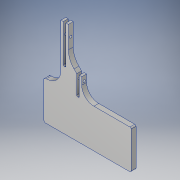
# Autodesk Inventor part: 2BarClawPaddle
Saved by Autodesk Inventor 2017 (Build 210142000, 142)
## iProperties
Created: 2017-09-30
Part Number: 2BarClawPaddle
Material: Aluminum 6061
Document SubType Name: Modeling
Designer: User
Density: 2.7 g/cm^3
Appearance: Aluminum - Flat
Mass: 78.5401 g
Surface Area: 128.456 cm^2
Volume: 29.0889 cm^3
Author: User
Autodesk Inventor part; units mm, degrees
ref_plane "YZ Plane" through (0, 0, 0) normal (1, 0, 0) x (0, 1, 0)
ref_plane "XZ Plane" through (0, 0, 0) normal (0, 1, 0) x (-1, 0, 0)
ref_plane "XY Plane" through (0, 0, 0) normal (0, 0, 1) x (1, 0, 0)
sketch "Sketch1" plane through (0, 0, 0) normal (0, 0, 1) x (1, 0, 0)
  line L0 (0, 0) -> (114.3, 0)
  line L1 (0, 0) -> (0, -50.8)
  line L2 (0, -50.8) -> (114.3, -50.8)
  line L3 (114.3, -50.8) -> (114.3, 0)
  dimension "d1" = 114.3
  dimension "d2" = 50.8
  dimension "d3" = 114.3
  constraints: 8 end point, 1 horizontal, 1 perpendicular, 1 vertical
  measures "d1" distance of L0.start L0.end
  measures "d2" distance of L0.start L1.end
  measures "d3" distance of L1.end L2.end
extrude "Extrusion1" add sketch "Sketch1" along normal blind 3.175
sketch "Sketch2" plane through (0, 0, 0) normal (0, 1, 0) x (1, 0, 0)
  line L0 (114.3, -3.175) -> (0, -3.175) projected
  line L1 (25.3873, -1.5875) -> (25.3873, 0)
  line L2 (25.3873, -3.175) -> (25.3873, -1.5875)
  line L3 (28.7401, -1.5875) -> (28.7401, -3.175)
  line L4 (28.7401, -1.5875) -> (28.7401, 0)
  line L5 (25.3873, -3.175) -> (22.2123, -3.175)
  line L6 (22.2123, -3.175) -> (22.2123, 3.175)
  line L7 (28.7401, -3.175) -> (31.9151, -3.175)
  line L8 (31.9151, -3.175) -> (31.9151, 3.175)
  line L9 (25.3873, 0) -> (25.3873, 3.175)
  line L10 (25.3873, 3.175) -> (22.2123, 3.175)
  line L11 (31.9151, 3.175) -> (28.7401, 3.175)
  line L12 (28.7401, 3.175) -> (28.7401, 0)
  point P0 (27.0637, -1.5875)
  dimension "d7" = 1.6764
  dimension "d8" = 1.6764
  dimension "d9" = 3.175
  dimension "d10" = 6.35
  dimension "d11" = 3.175
  constraints: 24 end point, 7 point on line, 4 perpendicular, 1 collinear, 1 vertical
  measures "d7" distance of point (27.064, -1.587) L3.start
  measures "d8" distance of point (27.064, -1.587) L1.start
  measures "d9" distance of L2.start L5.end
  measures "d10" distance of L5.end L6.end
  measures "d11" distance of L3.end L7.end
sketch "Sketch3" plane through (0, 0, 0) normal (0, 0, -1) x (-1, 0, 0)
  line L0 (-114.3, 0) -> (0, 0) projected
  line L1 (0, -50.8) -> (-114.3, -50.8) projected
  line L2 (0, 0) -> (-114.3, 0)
  line L3 (-114.3, 0) -> (-114.3, -50.8)
  line L4 (-114.3, -50.8) -> (0, -50.8)
  line L5 (0, -50.8) -> (0, 0)
  constraints: 8 end point, 2 parallel, 1 horizontal, 1 perpendicular
extrude "Extrusion2" add sketch "Sketch3" along normal blind 3.175
extrude "Extrusion3" add sketch "Sketch2" along normal blind 76.2 contours L0 L3 L4 L12 L11 L8
extrude "Extrusion4" add sketch "Sketch2" along normal blind 76.2 contours L0 L6 L10 L9 L1 L2
sketch "Sketch4" plane through (31.9151, 0, 3.175) normal (1, 0, 0) x (0, 0, -1)
  line L0 (3.175, 0) -> (3.175, 19.05)
  circle A0 centre (3.175, 19.05) radius 1.5875
  dimension "d18" = 19.05
  dimension "d19" = 3.175
  constraints: 2 end point, 1 centre point, 1 coincident, 1 vertical
  measures "d18" distance of L0.start L0.end
  measures "d19" diameter of A0
extrude "Extrusion5" cut sketch "Sketch4" along normal mid plane 50.8
sketch "Sketch5" plane through (31.9151, 0, 3.175) normal (1, 0, 0) x (0, 0, -1)
  circle A0 centre (3.175, 19.05) radius 1.5875 projected
  line L0 (3.175, 19.05) -> (3.175, 60.706)
  circle A1 centre (3.175, 60.706) radius 1.5875
  point P0 (3.175, 0)
  dimension "d22" = 41.656
  dimension "d23" = 3.175
  constraints: 2 end point, 1 centre point, 1 coincident, 1 vertical
  measures "d22" distance of L0.start L0.end
  measures "d23" diameter of A1
extrude "Extrusion6" cut sketch "Sketch5" against normal blind 50.8 contours A1
sketch "Sketch6" plane through (25.3873, 0, 3.175) normal (1, 0, 0) x (0, 0, -1)
  point P0 (3.175, 0)
sketch "Sketch7" plane through (0, 0, 3.175) normal (0, 0, 1) x (1, 0, 0)
  point P0 (0, 0)
sketch "Sketch8" plane through (0, 0, 3.175) normal (0, 0, 1) x (1, 0, 0)
  line L0 (38.0873, 0) -> (41.2623, 0)
  line L1 (41.2623, 0) -> (41.2623, 22.5425)
  line L2 (38.0873, 0) -> (38.0873, 22.5425)
  line L3 (38.0873, 22.5425) -> (41.2623, 22.5425)
  line L4 (38.0873, 22.5425) -> (31.9151, 22.5425)
  line L5 (31.9151, 0) -> (31.9151, 76.2) projected
  line L6 (41.2623, 22.5425) -> (41.2623, 25.7175)
  line L7 (41.2623, 25.7175) -> (31.9151, 25.7175)
  point P0 (0, 0)
  dimension "d30" = 3.175
  dimension "d34" = 3.175
  constraints: 14 end point, 3 perpendicular, 2 horizontal, 2 point on line, 1 vertical
  measures "d30" distance of L0.start L0.end
  measures "d34" distance of L1.end L6.end
sketch "Sketch9" plane through (0, 0, 3.175) normal (0, 0, 1) x (1, 0, 0)
  line L0 (41.2623, 25.7175) -> (41.2623, 0) projected
  line L1 (31.9151, 0) -> (114.3, 0) projected
  line L2 (44.6151, 0) -> (44.6151, 25.6324)
  line L3 (44.6151, 25.6324) -> (47.7901, 25.6324)
  line L4 (47.7901, 0) -> (47.7901, 25.6324)
  line L5 (44.6151, 0) -> (47.7901, 0)
  point P0 (0, 0)
  dimension "d35" = 3.3528
  dimension "d36" = 3.175
  constraints: 8 end point, 2 perpendicular, 2 point on line, 1 collinear, 1 vertical
  measures "d35" distance of L0.end L2.start
  measures "d36" distance of L2.end L3.end
sketch "Sketch12" plane through (0, 0, 3.175) normal (0, 0, 1) x (1, 0, 0)
  line L0 (44.6151, 0) -> (44.6151, 25.6324) projected
  line L1 (44.6151, 0) -> (46.3169, 0)
  line L2 (46.3169, 0) -> (49.4919, 0)
  line L3 (25.3873, 0) -> (114.3, 0) projected
  line L4 (49.4919, 0) -> (49.4919, 25.6324)
  line L5 (49.4919, 25.6324) -> (46.3169, 25.6324)
  line L6 (46.3169, 25.6324) -> (46.3169, 0)
  point P0 (0, 0)
  point P1 (47.7901, 0)
  point P2 (41.2623, 0)
  dimension "d44" = 1.7018
  dimension "d45" = 3.175
  constraints: 10 end point, 3 perpendicular, 1 horizontal, 1 point on line
  measures "d44" distance of L0.start L1.end
  measures "d45" distance of L1.end L2.end
extrude "Extrusion11" add sketch "Sketch12" against normal blind 6.35
sketch "Sketch13" plane through (0, 0, 3.175) normal (0, 0, 1) x (1, 0, 0)
  line L0 (38.0873, 22.5425) -> (38.0873, 0) projected
  line L1 (38.0873, 0) -> (39.7891, 0)
  line L2 (39.7891, 0) -> (42.9641, 0)
  line L3 (46.3169, 0) -> (31.9151, 0) projected
  line L4 (39.7891, 0) -> (39.7891, 25.7175)
  line L5 (41.2623, 25.7175) -> (31.9151, 25.7175) projected
  line L6 (42.9641, 0) -> (42.9641, 25.7175)
  line L7 (42.9641, 25.7175) -> (39.7891, 25.7175)
  point P0 (0, 0)
  point P1 (41.2623, 0)
  dimension "d48" = 1.7018
  dimension "d49" = 3.175
  constraints: 10 end point, 2 point on line, 2 vertical, 1 horizontal, 1 perpendicular
  measures "d48" distance of L0.end L1.end
  measures "d49" distance of L1.end L2.end
extrude "Extrusion12" add sketch "Sketch13" against normal blind 6.35
sketch "Sketch14" plane through (0, 0, 3.175) normal (0, 0, 1) x (1, 0, 0)
  line L0 (39.7891, 25.7175) -> (42.9641, 25.7175) projected
  line L1 (39.7891, 25.7175) -> (39.7891, 22.5425)
  line L2 (39.7891, 25.7175) -> (39.7891, 0) projected
  line L3 (39.7891, 22.5425) -> (31.9151, 22.5425)
  line L4 (39.7891, 25.7175) -> (50.9246, 25.7175) construction
  line L5 (42.9641, 25.7175) -> (56.7757, 25.7175) construction
  line L6 (31.9151, 0) -> (31.9151, 76.2) projected
  line L7 (31.9151, 36.7665) -> (42.9641, 25.7175)
  line L8 (31.9151, 36.7665) -> (31.9151, 22.5425)
  line L9 (42.9641, 25.7175) -> (39.7891, 25.7175) projected
  line L10 (39.7891, 25.7175) -> (42.9641, 25.7175)
  point P0 (0, 0)
  dimension "d52" = 3.175
  constraints: 14 end point, 2 collinear, 2 horizontal, 2 point on line, 1 perpendicular
  measures "d52" distance of L0.start L1.end
extrude "Extrusion13" add sketch "Sketch14" against normal blind 6.35
sketch "Sketch15" plane through (22.2123, 0, -3.175) normal (-1, 0, 0) x (0, 0, 1)
  circle A0 centre (3.175, 19.05) radius 1.5875 projected
  circle A1 centre (3.175, 19.05) radius 1.5875
  point P0 (3.175, 0)
  constraints: 1 centre point, 1 coincident
extrude "Extrusion14" cut sketch "Sketch15" against normal blind 50.8
sketch "Sketch16" plane through (0, 0, 3.175) normal (0, 0, 1) x (1, 0, 0)
  line L0 (31.9151, 36.7665) -> (42.9641, 25.7175) projected
  line L1 (42.9641, 25.7175) -> (22.2123, 25.7175)
  line L2 (22.2123, 0) -> (22.2123, 76.2) projected
  line L3 (42.9641, 25.7175) -> (42.9641, 0) projected
  line L4 (42.9641, 0) -> (22.2123, 0)
  line L5 (22.2123, 0) -> (22.2123, 25.7175)
  line L6 (42.9641, 25.7175) -> (42.9641, 0)
  point P0 (0, 0)
  constraints: 8 end point, 2 horizontal, 1 parallel, 1 perpendicular, 1 point on line
extrude "Extrusion15" add sketch "Sketch16" against normal blind 6.35
sketch "Sketch17" plane through (49.4919, 0, 3.175) normal (1, 0, 0) x (0, 0, -1)
  circle A0 centre (3.175, 19.05) radius 1.5875 projected
  circle A1 centre (3.175, 19.05) radius 1.5875
  point P0 (3.175, 0)
  constraints: 1 centre point, 1 coincident
extrude "Extrusion16" cut sketch "Sketch17" against normal blind 12.7
fillet "Fillet1" radius 1.5875 2 edges at (42.9641, 0, 0) (46.3169, 0, 0)
fillet "Fillet3" radius 25.4 1 edges at (31.9151, 36.7665, 0)
fillet "Fillet4" radius 1.5875 6 edges at (0, 0, 0) (0, -50.8, 0) (114.3, -50.8, 0) (114.3, 0, 0) (25.3873, 25.7175, 0) (28.7401, 25.7175, 0)
fillet "Fillet5" radius 15.875 1 edges at (49.4919, 0, 0)
fillet "Fillet6" radius 19.05 1 edges at (22.2123, 0, 0)
body "Solid1"
